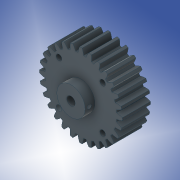
# Autodesk Inventor part: BA011
Saved by Autodesk Inventor 2017 (Build 210142000, 142)
## iProperties
Created: 2017-06-23
Part Number: BA011
Material: ABS Plastic
Document SubType Name: Modeling
Designer: zallen
Density: 1.06 g/cm^3
Appearance: CR Dark Blue
Author: zallen
Autodesk Inventor part; units mm, degrees
ref_plane "YZ Plane" through (0, 0, 0) normal (1, 0, 0) x (0, 1, 0)
ref_plane "XZ Plane" through (0, 0, 0) normal (0, 1, 0) x (-1, 0, 0)
ref_plane "XY Plane" through (0, 0, 0) normal (0, 0, 1) x (1, 0, 0)
sketch "Sketch1" plane through (0, 0, 0) normal (0, 0, 1) x (1, 0, 0)
  circle A0 centre (0, 0) radius 3
  circle A1 centre (0, 0) radius 25.5
  dimension "d0" = 6
  dimension "d1" = 51
  constraints: 2 centre point, 2 coincident
  measures "d0" diameter of A0
  measures "d1" diameter of A1
extrude "Extrusion1" add sketch "Sketch1" along normal blind 20
sketch "Sketch2" plane through (0, 0, 20) normal (0, 0, 1) x (1, 0, 0)
  line L0 (0, 0) -> (50, 0) construction
  circle A0 centre (0, 0) radius 25.5 projected
  circle A1 centre (0, 0) radius 25.5 projected
  arc A2 (29.4214, 0.9) -> (25.4214, 2) centre (23.4823, -12.8741) ccw
  arc A3 (29.4214, -0.9) -> (29.4214, 0.9) centre (9.4417, 0) ccw
  arc A4 (25.4214, -2) -> (29.4214, -0.9) centre (23.4823, 12.8741) ccw
  arc A5 (25.4214, -2) -> (25.4214, 2) centre (0, 0) ccw
  arc A6 (28.4835, 7.4243) -> (24.339, 7.6067) centre (25.7583, -7.326) ccw
  arc A7 (28.8841, 5.6695) -> (28.4835, 7.4243) centre (9.205, 2.101) ccw
  arc A8 (25.2291, 3.7069) -> (28.8841, 5.6695) centre (20.0288, 17.7767) ccw
  arc A9 (25.2291, 3.7069) -> (24.339, 7.6067) centre (0, 0) ccw
  arc A10 (26.1173, 13.5764) -> (22.0362, 12.8319) centre (26.7427, -1.4106) ccw
  arc A11 (26.8983, 11.9546) -> (26.1173, 13.5764) centre (8.5067, 4.0966) ccw
  arc A12 (23.7717, 9.228) -> (26.8983, 11.9546) centre (15.571, 21.7878) ccw
  arc A13 (23.7717, 9.228) -> (22.0362, 12.8319) centre (0, 0) ccw
  arc A14 (22.4415, 19.0476) -> (18.6283, 17.4137) centre (26.3861, 4.5756) ccw
  arc A15 (23.5638, 17.6403) -> (22.4415, 19.0476) centre (7.3818, 5.8868) ccw
  arc A16 (21.1223, 14.2864) -> (23.5638, 17.6403) centre (10.3323, 24.7064) ccw
  arc A17 (21.1223, 14.2864) -> (18.6283, 17.4137) centre (0, 0) ccw
  arc A18 (17.6403, 23.5638) -> (14.2864, 21.1223) centre (24.7064, 10.3323) ccw
  arc A19 (19.0476, 22.4415) -> (17.6403, 23.5638) centre (5.8868, 7.3818) ccw
  arc A20 (17.4137, 18.6283) -> (19.0476, 22.4415) centre (4.5756, 26.3861) ccw
  arc A21 (17.4137, 18.6283) -> (14.2864, 21.1223) centre (0, 0) ccw
  arc A22 (11.9546, 26.8983) -> (9.228, 23.7717) centre (21.7878, 15.571) ccw
  arc A23 (13.5764, 26.1173) -> (11.9546, 26.8983) centre (4.0966, 8.5067) ccw
  arc A24 (12.8319, 22.0362) -> (13.5764, 26.1173) centre (-1.4106, 26.7427) ccw
  arc A25 (12.8319, 22.0362) -> (9.228, 23.7717) centre (0, 0) ccw
  arc A26 (5.6695, 28.8841) -> (3.7069, 25.2291) centre (17.7767, 20.0288) ccw
  arc A27 (7.4243, 28.4835) -> (5.6695, 28.8841) centre (2.101, 9.205) ccw
  arc A28 (7.6067, 24.339) -> (7.4243, 28.4835) centre (-7.326, 25.7583) ccw
  arc A29 (7.6067, 24.339) -> (3.7069, 25.2291) centre (0, 0) ccw
  arc A30 (-0.9, 29.4214) -> (-2, 25.4214) centre (12.8741, 23.4823) ccw
  arc A31 (0.9, 29.4214) -> (-0.9, 29.4214) centre (0, 9.4417) ccw
  arc A32 (2, 25.4214) -> (0.9, 29.4214) centre (-12.8741, 23.4823) ccw
  arc A33 (2, 25.4214) -> (-2, 25.4214) centre (0, 0) ccw
  arc A34 (-7.4243, 28.4835) -> (-7.6067, 24.339) centre (7.326, 25.7583) ccw
  arc A35 (-5.6695, 28.8841) -> (-7.4243, 28.4835) centre (-2.101, 9.205) ccw
  arc A36 (-3.7069, 25.2291) -> (-5.6695, 28.8841) centre (-17.7767, 20.0288) ccw
  arc A37 (-3.7069, 25.2291) -> (-7.6067, 24.339) centre (0, 0) ccw
  arc A38 (-13.5764, 26.1173) -> (-12.8319, 22.0362) centre (1.4106, 26.7427) ccw
  arc A39 (-11.9546, 26.8983) -> (-13.5764, 26.1173) centre (-4.0966, 8.5067) ccw
  arc A40 (-9.228, 23.7717) -> (-11.9546, 26.8983) centre (-21.7878, 15.571) ccw
  arc A41 (-9.228, 23.7717) -> (-12.8319, 22.0362) centre (0, 0) ccw
  arc A42 (-19.0476, 22.4415) -> (-17.4137, 18.6283) centre (-4.5756, 26.3861) ccw
  arc A43 (-17.6403, 23.5638) -> (-19.0476, 22.4415) centre (-5.8868, 7.3818) ccw
  arc A44 (-14.2864, 21.1223) -> (-17.6403, 23.5638) centre (-24.7064, 10.3323) ccw
  arc A45 (-14.2864, 21.1223) -> (-17.4137, 18.6283) centre (0, 0) ccw
  arc A46 (-23.5638, 17.6403) -> (-21.1223, 14.2864) centre (-10.3323, 24.7064) ccw
  arc A47 (-22.4415, 19.0476) -> (-23.5638, 17.6403) centre (-7.3818, 5.8868) ccw
  arc A48 (-18.6283, 17.4137) -> (-22.4415, 19.0476) centre (-26.3861, 4.5756) ccw
  arc A49 (-18.6283, 17.4137) -> (-21.1223, 14.2864) centre (0, 0) ccw
  arc A50 (-26.8983, 11.9546) -> (-23.7717, 9.228) centre (-15.571, 21.7878) ccw
  arc A51 (-26.1173, 13.5764) -> (-26.8983, 11.9546) centre (-8.5067, 4.0966) ccw
  arc A52 (-22.0362, 12.8319) -> (-26.1173, 13.5764) centre (-26.7427, -1.4106) ccw
  arc A53 (-22.0362, 12.8319) -> (-23.7717, 9.228) centre (0, 0) ccw
  arc A54 (-28.8841, 5.6695) -> (-25.2291, 3.7069) centre (-20.0288, 17.7767) ccw
  arc A55 (-28.4835, 7.4243) -> (-28.8841, 5.6695) centre (-9.205, 2.101) ccw
  arc A56 (-24.339, 7.6067) -> (-28.4835, 7.4243) centre (-25.7583, -7.326) ccw
  arc A57 (-24.339, 7.6067) -> (-25.2291, 3.7069) centre (0, 0) ccw
  arc A58 (-29.4214, -0.9) -> (-25.4214, -2) centre (-23.4823, 12.8741) ccw
  arc A59 (-29.4214, 0.9) -> (-29.4214, -0.9) centre (-9.4417, 0) ccw
  arc A60 (-25.4214, 2) -> (-29.4214, 0.9) centre (-23.4823, -12.8741) ccw
  arc A61 (-25.4214, 2) -> (-25.4214, -2) centre (0, 0) ccw
  arc A62 (-28.4835, -7.4243) -> (-24.339, -7.6067) centre (-25.7583, 7.326) ccw
  arc A63 (-28.8841, -5.6695) -> (-28.4835, -7.4243) centre (-9.205, -2.101) ccw
  arc A64 (-25.2291, -3.7069) -> (-28.8841, -5.6695) centre (-20.0288, -17.7767) ccw
  arc A65 (-25.2291, -3.7069) -> (-24.339, -7.6067) centre (0, 0) ccw
  arc A66 (-26.1173, -13.5764) -> (-22.0362, -12.8319) centre (-26.7427, 1.4106) ccw
  arc A67 (-26.8983, -11.9546) -> (-26.1173, -13.5764) centre (-8.5067, -4.0966) ccw
  arc A68 (-23.7717, -9.228) -> (-26.8983, -11.9546) centre (-15.571, -21.7878) ccw
  arc A69 (-23.7717, -9.228) -> (-22.0362, -12.8319) centre (0, 0) ccw
  arc A70 (-22.4415, -19.0476) -> (-18.6283, -17.4137) centre (-26.3861, -4.5756) ccw
  arc A71 (-23.5638, -17.6403) -> (-22.4415, -19.0476) centre (-7.3818, -5.8868) ccw
  arc A72 (-21.1223, -14.2864) -> (-23.5638, -17.6403) centre (-10.3323, -24.7064) ccw
  arc A73 (-21.1223, -14.2864) -> (-18.6283, -17.4137) centre (0, 0) ccw
  arc A74 (-17.6403, -23.5638) -> (-14.2864, -21.1223) centre (-24.7064, -10.3323) ccw
  arc A75 (-19.0476, -22.4415) -> (-17.6403, -23.5638) centre (-5.8868, -7.3818) ccw
  arc A76 (-17.4137, -18.6283) -> (-19.0476, -22.4415) centre (-4.5756, -26.3861) ccw
  arc A77 (-17.4137, -18.6283) -> (-14.2864, -21.1223) centre (0, 0) ccw
  arc A78 (-11.9546, -26.8983) -> (-9.228, -23.7717) centre (-21.7878, -15.571) ccw
  arc A79 (-13.5764, -26.1173) -> (-11.9546, -26.8983) centre (-4.0966, -8.5067) ccw
  arc A80 (-12.8319, -22.0362) -> (-13.5764, -26.1173) centre (1.4106, -26.7427) ccw
  arc A81 (-12.8319, -22.0362) -> (-9.228, -23.7717) centre (0, 0) ccw
  arc A82 (-5.6695, -28.8841) -> (-3.7069, -25.2291) centre (-17.7767, -20.0288) ccw
  arc A83 (-7.4243, -28.4835) -> (-5.6695, -28.8841) centre (-2.101, -9.205) ccw
  arc A84 (-7.6067, -24.339) -> (-7.4243, -28.4835) centre (7.326, -25.7583) ccw
  arc A85 (-7.6067, -24.339) -> (-3.7069, -25.2291) centre (0, 0) ccw
  arc A86 (0.9, -29.4214) -> (2, -25.4214) centre (-12.8741, -23.4823) ccw
  arc A87 (-0.9, -29.4214) -> (0.9, -29.4214) centre (0, -9.4417) ccw
  arc A88 (-2, -25.4214) -> (-0.9, -29.4214) centre (12.8741, -23.4823) ccw
  arc A89 (-2, -25.4214) -> (2, -25.4214) centre (0, 0) ccw
  arc A90 (7.4243, -28.4835) -> (7.6067, -24.339) centre (-7.326, -25.7583) ccw
  arc A91 (5.6695, -28.8841) -> (7.4243, -28.4835) centre (2.101, -9.205) ccw
  arc A92 (3.7069, -25.2291) -> (5.6695, -28.8841) centre (17.7767, -20.0288) ccw
  arc A93 (3.7069, -25.2291) -> (7.6067, -24.339) centre (0, 0) ccw
  arc A94 (13.5764, -26.1173) -> (12.8319, -22.0362) centre (-1.4106, -26.7427) ccw
  arc A95 (11.9546, -26.8983) -> (13.5764, -26.1173) centre (4.0966, -8.5067) ccw
  arc A96 (9.228, -23.7717) -> (11.9546, -26.8983) centre (21.7878, -15.571) ccw
  arc A97 (9.228, -23.7717) -> (12.8319, -22.0362) centre (0, 0) ccw
  arc A98 (19.0476, -22.4415) -> (17.4137, -18.6283) centre (4.5756, -26.3861) ccw
  arc A99 (17.6403, -23.5638) -> (19.0476, -22.4415) centre (5.8868, -7.3818) ccw
  arc A100 (14.2864, -21.1223) -> (17.6403, -23.5638) centre (24.7064, -10.3323) ccw
  arc A101 (14.2864, -21.1223) -> (17.4137, -18.6283) centre (0, 0) ccw
  arc A102 (23.5638, -17.6403) -> (21.1223, -14.2864) centre (10.3323, -24.7064) ccw
  arc A103 (22.4415, -19.0476) -> (23.5638, -17.6403) centre (7.3818, -5.8868) ccw
  arc A104 (18.6283, -17.4137) -> (22.4415, -19.0476) centre (26.3861, -4.5756) ccw
  arc A105 (18.6283, -17.4137) -> (21.1223, -14.2864) centre (0, 0) ccw
  arc A106 (26.8983, -11.9546) -> (23.7717, -9.228) centre (15.571, -21.7878) ccw
  arc A107 (26.1173, -13.5764) -> (26.8983, -11.9546) centre (8.5067, -4.0966) ccw
  arc A108 (22.0362, -12.8319) -> (26.1173, -13.5764) centre (26.7427, 1.4106) ccw
  arc A109 (22.0362, -12.8319) -> (23.7717, -9.228) centre (0, 0) ccw
  arc A110 (28.8841, -5.6695) -> (25.2291, -3.7069) centre (20.0288, -17.7767) ccw
  arc A111 (28.4835, -7.4243) -> (28.8841, -5.6695) centre (9.205, -2.101) ccw
  arc A112 (24.339, -7.6067) -> (28.4835, -7.4243) centre (25.7583, 7.326) ccw
  arc A113 (24.339, -7.6067) -> (25.2291, -3.7069) centre (0, 0) ccw
  point P0 (29.4417, 0)
  point P1 (28.7035, 6.5514)
  point P2 (26.5261, 12.7743)
  point P3 (23.0185, 18.3566)
  point P4 (18.3566, 23.0185)
  point P5 (12.7743, 26.5261)
  point P6 (6.5514, 28.7035)
  point P7 (0, 29.4417)
  point P8 (-6.5514, 28.7035)
  point P9 (-12.7743, 26.5261)
  point P10 (-18.3566, 23.0185)
  point P11 (-23.0185, 18.3566)
  point P12 (-26.5261, 12.7743)
  point P13 (-28.7035, 6.5514)
  point P14 (-29.4417, 0)
  point P15 (-28.7035, -6.5514)
  point P16 (-26.5261, -12.7743)
  point P17 (-23.0185, -18.3566)
  point P18 (-18.3566, -23.0185)
  point P19 (-12.7743, -26.5261)
  point P20 (-6.5514, -28.7035)
  point P21 (0, -29.4417)
  point P22 (6.5514, -28.7035)
  point P23 (12.7743, -26.5261)
  point P24 (18.3566, -23.0185)
  point P25 (23.0185, -18.3566)
  point P26 (26.5261, -12.7743)
  point P27 (28.7035, -6.5514)
  dimension "d4" = 50
  dimension "d5" = 15
  dimension "d6" = 4
  dimension "d7" = 2
  dimension "d8" = 20
  dimension "d10" = 15
  dimension "d11" = 4
  dimension "d12" = 2
  dimension "d15" = 360
  dimension "d34" = 1.8
  constraints: 229 point on circle, 112 centre point, 3 coincident, 2 end point, 1 horizontal, 1 point on line, 363 other
  measures "d4" distance of L0.start L0.end
  measures "d5" radius of A2
  measures "d6" horizontal distance of A2.start A0.start
  measures "d7" distance from line of L0 A0.start
  measures "d8" radius of A3
  measures "d10" radius of A4
  measures "d11" horizontal distance of A3.start A0.end
  measures "d12" distance from line of L0 A0.end
  measures "d34" distance of A3.start A2.start
extrude "Extrusion2" add sketch "Sketch2" against normal blind 20 contours A0 A2 A3 A4 | A0 A6 A7 A8 | A110 A111 A112 A0 | A0 A10 A11 A12 | A106 A107 A108 A0 | A0 A14 A15 A16 | A102 A103 A104 A0 | A0 A18 A19 A20 | A98 A99 A100 A0 | A0 A22 A23 A24 | A94 A95 A96 A0 | A0 A26 A27 A28 | A90 A91 A92 A0 | A0 A30 A31 A32 | A86 A87 A88 A0 | A0 A34 A35 A36 | A82 A83 A84 A0 | A0 A38 A39 A40 | A78 A79 A80 A0 | A0 A42 A43 A44 | A74 A75 A76 A0 | A0 A46 A47 A48 | A70 A71 A72 A0 | A0 A50 A51 A52 | A66 A67 A68 A0 | A0 A54 A55 A56 | A62 A63 A64 A0 | A0 A58 A59 A60
sketch "Sketch3" plane through (0, 0, 20) normal (0, 0, 1) x (1, 0, 0)
  circle A0 centre (0, 0) radius 10
  circle A1 centre (0, 0) radius 3 projected
  dimension "d19" = 20
  constraints: 1 centre point, 1 coincident
  measures "d19" diameter of A0
extrude "Extrusion3" add sketch "Sketch3" along normal blind 7
sketch "Sketch4" plane through (0, 0, 20) normal (0, 0, 1) x (1, 0, 0)
  line L0 (-15.5, -15.5) -> (15.5, -15.5) construction
  line L1 (15.5, -15.5) -> (15.5, 15.5) construction
  line L2 (15.5, 15.5) -> (-15.5, 15.5) construction
  line L3 (-15.5, 15.5) -> (-15.5, -15.5) construction
  circle A0 centre (-15.5, 15.5) radius 2
  circle A1 centre (15.5, 15.5) radius 2
  circle A2 centre (15.5, -15.5) radius 2
  circle A3 centre (-15.5, -15.5) radius 2
  point P0 (0, 0)
  point P1 (-15.5, 0)
  point P2 (0, 15.5)
  dimension "d22" = 31
  dimension "d23" = 31
  dimension "d24" = 4
  dimension "d25" = 4
  dimension "d26" = 4
  dimension "d27" = 4
  constraints: 8 end point, 4 centre point, 4 coincident, 2 midpoint, 2 parallel, 1 horizontal, 1 horizontal alignment, 1 perpendicular, 1 vertical alignment
  measures "d22" distance of L2.end L1.end
  measures "d23" distance of L1.end L0.end
  measures "d24" diameter of A0
  measures "d25" diameter of A1
  measures "d26" diameter of A2
  measures "d27" diameter of A3
extrude "Extrusion4" cut sketch "Sketch4" against normal through all
sketch "Sketch5" plane through (0, 0, 0) normal (1, 0, 0) x (0, 1, 0)
  circle A0 centre (0, 24) radius 1.5
  line L0 (10, 27) -> (-10, 27) projected
  point P0 (0, 0)
  dimension "d30" = 3
  dimension "d31" = 3
  constraints: 1 centre point
  measures "d30" diameter of A0
  measures "d31" distance from line of L0 A0.centre
extrude "Extrusion5" cut sketch "Sketch5" along normal through all
body "Solid1"
